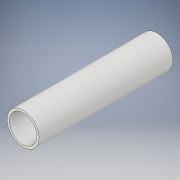
# Autodesk Inventor part: 2_5-inch schedule 40
Saved by Autodesk Inventor 2018.2 (Build 222227000, 227)
## iProperties
Created: 2018-01-07
Part Number: 2_5-inch schedule 40
Material: PVC-Piping
Document SubType Name: Modeling
Designer: steele
Density: 1.4 g/cm^3
Appearance: Smooth - White
Author: steele
Autodesk Inventor part; units mm, degrees
ref_plane "YZ Plane" through (0, 0, 0) normal (1, 0, 0) x (0, 1, 0)
ref_plane "XZ Plane" through (0, 0, 0) normal (0, 1, 0) x (-1, 0, 0)
ref_plane "XY Plane" through (0, 0, 0) normal (0, 0, 1) x (1, 0, 0)
sketch "Sketch1" plane through (0, 0, 0) normal (0, 0, 1) x (1, 0, 0)
  circle A0 centre (0, 0) radius 31.3563
  circle A1 centre (0, 0) radius 36.5125
  dimension "d0" = 62.7126
  dimension "d1" = 73.025
  constraints: 2 centre point, 2 coincident
  measures "d0" diameter of A0
  measures "d1" diameter of A1
extrude "Extrusion1" add sketch "Sketch1" against normal blind 304.8
body "Solid1"
